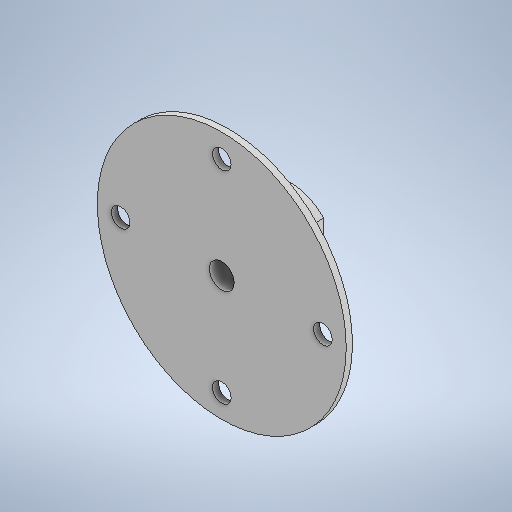
# Autodesk Inventor part: Sprocket Adapter
Saved by Autodesk Inventor 2025.2 (Build 292293000, 293)
## iProperties
Created: 2025-03-23
Part Number: Sprocket Adapter
Material: Generic
Document SubType Name: Modeling
Designer: Mathias
Density: 1 g/cm^3
Appearance: Default
Author: Mathias
Autodesk Inventor part; units mm, degrees
ref_plane "YZ Plane" through (0, 0, 0) normal (1, 0, 0) x (0, 1, 0)
ref_plane "XZ Plane" through (0, 0, 0) normal (0, 1, 0) x (-1, 0, 0)
ref_plane "XY Plane" through (0, 0, 0) normal (0, 0, 1) x (1, 0, 0)
sketch "Sketch1" plane through (0, 0, 0) normal (0, 0, 1) x (1, 0, 0)
  circle A0 centre (0, 0) radius 40
  line L0 (0, 0) -> (32.5, 0)
  line L1 (0, 0) -> (0, 32.5)
  circle A1 centre (0, 32.5) radius 3
  circle A2 centre (32.5, 0) radius 3
  circle A3 centre (0, -32.5) radius 3
  circle A4 centre (-32.5, 0) radius 3
  circle A5 centre (0, 0) radius 4
  dimension "d0" = 80
  dimension "d1" = 32.5
  dimension "d2" = 32.5
  dimension "d3" = 6
  dimension "d4" = 6
  dimension "d5" = 8
  constraints: 6 centre point, 4 coincident, 4 end point, 2 symmetric about line, 1 horizontal, 1 vertical, 2 other
  measures "d0" diameter of A0
  measures "d1" distance of L0.start L0.end
  measures "d2" distance of L0.start L1.end
  measures "d3" diameter of A1
  measures "d4" diameter of A2
  measures "d5" diameter of A5
extrude "Extrusion1" add sketch "Sketch1" along normal blind 2
sketch "Sketch2" plane through (0, 0, 0) normal (0, 0, -1) x (-1, 0, 0)
  circle A0 centre (0, 0) radius 4 projected
  circle A1 centre (0, 0) radius 15
  dimension "d8" = 30
  constraints: 1 centre point, 1 coincident
  measures "d8" diameter of A1
extrude "Extrusion2" add sketch "Sketch2" along normal blind 20
sketch "Sketch3" plane through (0, 0, -20) normal (0, 0, -1) x (-1, 0, 0)
  circle A0 centre (0, 0) radius 15 projected
  line L0 (-10.7651, -10.4457) -> (-10.7651, 10.4457)
  circle A1 centre (0, 0) radius 15
  constraints: 2 end point, 2 point on circle, 1 coincident, 1 vertical, 3 other
extrude "Extrusion3" cut sketch "Sketch3" against normal blind 20 contours L0 A0 picked at (-11.4387, 2.6145)
sketch "Sketch4" plane through (10.7651, -10.4457, -20) normal (1, 0, 0) x (0, 0, -1)
  circle A0 centre (-11, 10.4457) radius 2.95
  point P0 (-20, 10.4457)
  dimension "d13" = 5.9
  constraints: 1 centre point
  measures "d13" diameter of A0
extrude "Extrusion4" cut sketch "Sketch4" against normal blind 11.75
thread "Thread1" size "M6x1" class "6H" standard "ISO Metric profile" length 19.85
body "Solid1"
